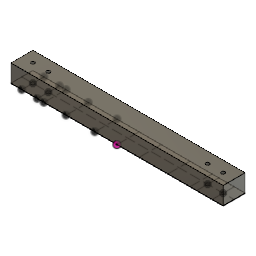
05part (Autodesk Fusion 360 design; units mm, degrees)
Autodesk Fusion 360 part; units mm, degrees
sketch "Sketch4" plane through (0, 0, 0) normal (0, 1, 0) x (1, 0, 0)
  line L0 (-240, 50) -> (240, 50)
  line L1 (240, 50) -> (240, 0)
  line L2 (240, 0) -> (-240, 0)
  line L3 (-240, 0) -> (-240, 50)
  line L4 (0, 50) -> (0, 0) construction
  line L5 (50, 50) -> (50, 0) construction
  line L6 (115, 50) -> (115, 0) construction
  line L7 (165, 50) -> (165, 0) construction
  line L8 (180, 50) -> (180, 0) construction
  line L9 (215, 50) -> (215, 0) construction
  line L10 (-115, 50) -> (-115, 0) construction
  line L11 (-50, 50) -> (-50, 0) construction
  line L12 (-165, 50) -> (-165, 0) construction
  line L13 (-180, 50) -> (-180, 0) construction
  line L14 (-215, 50) -> (-215, 0) construction
  line L15 (-240, 25) -> (240, 25) construction
  circle A0 centre (180, 25) radius 4
  circle A1 centre (215, 25) radius 4
  circle A2 centre (-180, 25) radius 4
  circle A3 centre (-215, 25) radius 4
  dimension "d6" = 480
  dimension "d7" = 50
  dimension "d8" = 100
  dimension "d9" = 50
  dimension "d10" = 330
  dimension "d11" = 25
  dimension "d12" = 35
  dimension "d13" = 8
  dimension "d14" = 8
  dimension "d15" = 8
  dimension "d16" = 8
  constraint horizontal L0
  constraint vertical L1
  constraint horizontal L2
  constraint vertical L3
  constraint midpoint L4.end L2
  constraint midpoint L0 L4.start
  constraint coincident L4.end origin
  constraint coincident L0 L5.start
  constraint coincident L2 L5.end
  constraint perpendicular L2 L5
  constraint coincident L0 L6.start
  constraint coincident L2 L6.end
  constraint perpendicular L2 L6
  constraint coincident L0 L7.start
  constraint coincident L2 L7.end
  constraint perpendicular L2 L7
  constraint coincident L0 L8.start
  constraint coincident L2 L8.end
  constraint perpendicular L2 L8
  constraint coincident L0 L9.start
  constraint coincident L2 L9.end
  constraint perpendicular L2 L9
  constraint symmetric L4 L5.start L11.start
  constraint symmetric L4 L5.end L11.end
  constraint symmetric L4 L6.start L10.start
  constraint symmetric L4 L6.end L10.end
  constraint symmetric L4 L7.start L12.start
  constraint symmetric L4 L7.end L12.end
  constraint symmetric L4 L8.start L13.start
  constraint symmetric L4 L8.end L13.end
  constraint symmetric L4 L9.start L14.start
  constraint symmetric L4 L9.end L14.end
  constraint midpoint L3 L15.start
  constraint midpoint L1 L15.end
  constraint midpoint L8 A0.centre
  constraint midpoint L9 A1.centre
  constraint midpoint L13 A2.centre
  constraint midpoint L14 A3.centre
  measures "d6" distance of L0.start L0.end
  measures "d7" distance of L0.start L2.end
  measures "d8" distance of L5 L11
  measures "d9" distance of L6 L7
  measures "d10" distance of L7 L12
  measures "d11" distance of L1 L9
  measures "d12" distance of L8 L9
  measures "d13" diameter of A0
  measures "d14" diameter of A1
  measures "d15" diameter of A2
  measures "d16" diameter of A3
extrude "Extrude1" add sketch "Sketch4" along normal blind 40
